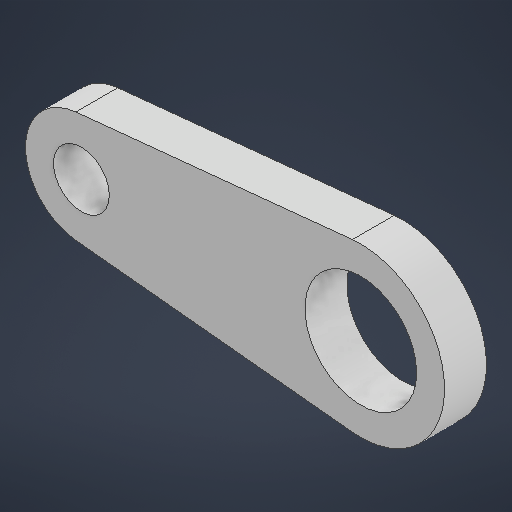
# Autodesk Inventor part: Part10
Saved by Autodesk Inventor 2026 (Build 300175050, 175E)
## iProperties
Created: 2026-03-26
Part Number: Part10
Material: Generic
Document SubType Name: Modeling
Designer: Administrator
Density: 1 g/cm^3
Appearance: Default
Author: Administrator
Autodesk Inventor part; units mm, degrees
ref_plane "YZ Plane" through (0, 0, 0) normal (1, 0, 0) x (0, 1, 0)
ref_plane "XZ Plane" through (0, 0, 0) normal (0, 1, 0) x (-1, 0, 0)
ref_plane "XY Plane" through (0, 0, 0) normal (0, 0, 1) x (1, 0, 0)
sketch "Sketch1" plane through (0, 0, 0) normal (0, 0, 1) x (1, 0, 0)
  line L0 (0, 0) -> (100, 0) construction
  circle A0 centre (100, 0) radius 20
  arc A1 (97, -29.8496) -> (97, 29.8496) centre (100, 0) ccw
  circle A2 centre (0, 0) radius 10
  arc A3 (-2, 19.8997) -> (-2, -19.8997) centre (0, 0) ccw
  line L1 (-2, 19.8997) -> (97, 29.8496)
  line L2 (-2, -19.8997) -> (97, -29.8496)
  dimension "d0" = 100
  dimension "d1" = 20
  dimension "d2" = 60
  dimension "d3" = 40
  dimension "d4" = 40
  constraints: 6 end point, 4 centre point, 4 coincident, 4 point on circle, 4 tangent, 1 horizontal
  measures "d0" distance of L0.start L0.end
  measures "d1" diameter of A2
  measures "d2" diameter of A1
  measures "d3" diameter of A0
  measures "d4" diameter of A3
extrude "Extrusion1" add sketch "Sketch1" along normal mid plane 15
body "Solid1"
